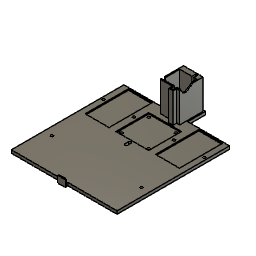
RobotBase (Autodesk Fusion 360 design; units mm, degrees)
Autodesk Fusion 360 part; units mm, degrees
sketch "Sketch2" plane through (0, 0, 0) normal (1, 0, 0) x (0, 0, -1)
  line L0 (0, 0) -> (0, 10)
  dimension "d53" = 10
  constraint coincident L0.start origin
  constraint vertical L0
  measures "d53" distance of L0.start L0.end
sketch "Sketch1" plane through (0, 0, 0) normal (0, 1, 0) x (1, 0, 0)
  line L0 (0, 0) -> (141.9, 0)
  line L1 (141.9, 0) -> (141.9, 151.05)
  line L2 (0, 151.05) -> (0, 0)
  line L3 (130.925, 43.6) -> (10.975, 43.6) construction
  circle A0 centre (10.975, 43.6) radius 1.75
  circle A1 centre (130.925, 43.6) radius 1.75
  line L4 (70.95, 0) -> (70.95, 43.6) construction
  line L5 (65.95, 0) -> (68.5, 0)
  line L6 (70.95, -2) -> (65.95, -2)
  line L7 (65.95, -2) -> (65.95, 0)
  line L8 (75.95, -2) -> (75.95, 0)
  line L9 (70.95, -2) -> (75.95, -2)
  line L10 (70.95, 43.6) -> (70.95, 85.6) construction
  line L11 (72.7, 88.1) -> (72.7, 83.1)
  line L12 (69.2, 83.1) -> (69.2, 88.1)
  arc A2 (72.7, 88.1) -> (69.2, 88.1) centre (70.95, 88.1) ccw
  arc A3 (69.2, 83.1) -> (72.7, 83.1) centre (70.95, 83.1) ccw
  line L13 (69.2, 85.6) -> (72.7, 85.6) construction
  line L14 (3.35, 120.45) -> (44.05, 120.45) construction
  circle A4 centre (3.35, 120.45) radius 1.75
  circle A5 centre (44.05, 120.45) radius 1.75
  line L15 (23.7, 151.05) -> (23.7, 120.45) construction
  line L16 (7.7, 149.45) -> (39.7, 149.45)
  line L17 (39.7, 149.45) -> (39.7, 91.45)
  line L18 (39.7, 91.45) -> (7.7, 91.45)
  line L19 (7.7, 91.45) -> (7.7, 149.45)
  line L20 (134.2, 91.45) -> (134.2, 149.45)
  line L21 (134.2, 149.45) -> (102.2, 149.45)
  line L22 (102.2, 149.45) -> (102.2, 91.45)
  circle A6 centre (138.55, 120.45) radius 1.75
  line L23 (102.2, 91.45) -> (134.2, 91.45)
  circle A7 centre (97.85, 120.45) radius 1.75
  line L24 (48.95, 135.45) -> (92.95, 135.45)
  line L25 (92.95, 135.45) -> (92.95, 91.45)
  line L26 (92.95, 91.45) -> (48.95, 91.45)
  line L27 (48.95, 91.45) -> (48.95, 135.45)
  line L28 (48.95, 113.45) -> (39.7, 113.45) construction
  line L29 (92.95, 113.45) -> (102.2, 113.45) construction
  circle A8 centre (52.7, 131.7) radius 1.75
  circle A9 centre (52.7, 95.2) radius 1.75
  circle A10 centre (89.2, 95.2) radius 1.75
  circle A11 centre (89.2, 131.7) radius 1.75
  line L30 (74.1, 142.05) -> (74.1, 137.05)
  line L31 (74.1, 173.25) -> (74.1, 168.25)
  line L32 (82.45, 143.65) -> (82.45, 166.65)
  line L33 (74.1, 173.25) -> (79.95, 173.25)
  line L34 (57.85, 142.05) -> (74.1, 142.05)
  line L35 (74.1, 168.25) -> (57.85, 168.25)
  line L36 (57.85, 142.05) -> (57.85, 168.25)
  line L37 (78.35, 138.65) -> (78.35, 143.65)
  line L38 (78.35, 166.65) -> (78.35, 171.65)
  line L39 (82.45, 166.65) -> (78.35, 166.65)
  line L40 (78.35, 143.65) -> (82.45, 143.65)
  line L41 (75.7, 166.65) -> (59.45, 166.65)
  line L42 (59.45, 166.65) -> (59.45, 143.65)
  line L43 (75.7, 171.65) -> (75.7, 166.65)
  line L44 (59.45, 143.65) -> (75.7, 143.65)
  line L45 (78.35, 171.65) -> (75.7, 171.65)
  line L46 (75.7, 138.65) -> (78.35, 138.65)
  line L47 (75.7, 143.65) -> (75.7, 138.65)
  line L48 (84.05, 142.05) -> (79.95, 142.05)
  line L49 (79.95, 137.05) -> (74.1, 137.05)
  line L50 (84.05, 168.25) -> (84.05, 142.05)
  line L51 (79.95, 142.05) -> (79.95, 137.05)
  line L52 (79.95, 168.25) -> (79.95, 173.25)
  line L53 (84.05, 168.25) -> (79.95, 168.25)
  line L54 (82.45, 155.15) -> (59.45, 155.15) construction
  line L55 (70.95, 155.15) -> (70.95, 135.45) construction
  line L56 (56.25, 151.05) -> (56.25, 174.85)
  line L57 (56.25, 174.85) -> (85.65, 174.85)
  line L58 (85.65, 174.85) -> (85.65, 151.05)
  line L59 (141.9, 151.05) -> (85.65, 151.05)
  line L60 (56.25, 151.05) -> (0, 151.05)
  line L61 (59.45, 143.65) -> (57.85, 143.65)
  line L62 (59.45, 147.65) -> (57.85, 147.65)
  line L63 (74.1, 173.25) -> (57.85, 173.25)
  line L64 (57.85, 173.25) -> (57.85, 168.25)
  line L65 (79.95, 173.25) -> (84.05, 173.25)
  line L66 (84.05, 173.25) -> (84.05, 168.25)
  line L67 (75.95, -2) -> (75.95, -3.6)
  line L68 (75.95, -3.6) -> (65.95, -3.6)
  line L69 (65.95, -3.6) -> (65.95, -2)
  point P0 (70.95, 113.45)
  point P1 (-289, 70)
  dimension "d1" = 141.9
  dimension "d2" = 151.05
  dimension "d3" = 119.95
  dimension "d4" = 3.5
  dimension "d6" = 5
  dimension "d8" = 43.6
  dimension "d9" = 42
  dimension "d10" = 3.5
  dimension "d11" = 5
  dimension "d12" = 40.7
  dimension "d13" = 3.5
  dimension "d14" = 3.35
  dimension "d15" = 30.6
  dimension "d16" = 58
  dimension "d17" = 1.6
  dimension "d18" = 32
  dimension "d19" = 16
  dimension "d20" = 44
  dimension "d23" = 44
  dimension "d24" = 3.35
  dimension "d25" = 3.5
  dimension "d26" = 3.75
  dimension "d27" = 3.75
  dimension "d28" = 22
  dimension "d29" = 22
  dimension "d31" = 360
  dimension "d32" = 4.9
  dimension "d33" = 4.9
  dimension "d34" = 1.6
  dimension "d35" = 1.6
  dimension "d36" = 1.6
  dimension "d37" = 1.6
  dimension "d38" = 1.6
  dimension "d39" = 1.6
  dimension "d40" = 1.6
  dimension "d41" = 1.6
  dimension "d42" = 1.6
  dimension "d43" = 1.6
  dimension "d44" = 1.6
  dimension "d45" = 1.6
  dimension "d47" = 5
  dimension "d48" = 23
  dimension "d49" = 23
  dimension "d50" = 4.1
  dimension "d51" = 6.75
  dimension "d54" = 1.6
  dimension "d55" = 1.6
  dimension "d56" = 1.6
  dimension "d57" = 1.6
  dimension "d58" = 4
  dimension "d80" = 2
  dimension "d81" = 1.6
  constraint horizontal L0
  constraint vertical L1
  constraint horizontal L59
  constraint vertical L2
  constraint coincident L0.start L2.end
  constraint perpendicular L2 L3
  constraint coincident L3.end A0.centre
  constraint coincident L3.start A1.centre
  constraint equal A0 A1
  constraint midpoint L0 L4.start
  constraint midpoint L3 L4.end
  constraint vertical L4
  constraint horizontal L5
  constraint horizontal L6
  constraint vertical L7
  constraint coincident L0 L5.start
  constraint coincident L4 L6.start
  constraint symmetric L4 L5.start L8.end
  constraint symmetric L4 L6.end L8.start
  constraint symmetric L4 L6.start L9.start
  constraint perpendicular L3 L10
  constraint vertical L11
  constraint vertical L12
  constraint tangent L12 A2
  constraint tangent L12 A3
  constraint tangent L11 A3
  constraint tangent L11 A2
  constraint coincident L10 A3.centre
  constraint midpoint L12 L13.start
  constraint midpoint L11 L13.end
  constraint coincident L10.end L13
  constraint horizontal L14
  constraint coincident L14.start A4.centre
  constraint coincident L14.end A5.centre
  constraint equal A4 A5
  constraint coincident L15.start L59
  constraint midpoint L14 L15.end
  constraint vertical L15
  constraint horizontal L16
  constraint vertical L17
  constraint horizontal L18
  constraint vertical L19
  constraint symmetric L10 A4 A6
  constraint symmetric L10 A5 A7
  constraint symmetric L10 L16.start L20.end
  constraint symmetric L10 L16.end L21.end
  constraint symmetric L10 L17.end L22.end
  constraint symmetric L10 L18.end L20.start
  constraint horizontal L24
  constraint vertical L25
  constraint horizontal L26
  constraint vertical L27
  constraint collinear L18 L26
  constraint midpoint L27 L28.start
  constraint coincident L17 L28.end
  constraint perpendicular L17 L28
  constraint midpoint L25 L29.start
  constraint coincident L22 L29.end
  constraint perpendicular L22 L29
  constraint equal L28 L29
  constraint perpendicular L31 L33
  constraint perpendicular L35 L36
  constraint perpendicular L50 L53
  constraint perpendicular L33 L52
  constraint perpendicular L48 L50
  constraint perpendicular L49 L51
  constraint perpendicular L34 L36
  constraint perpendicular L30 L49
  constraint coincident L32.start L40.end
  constraint collinear L37 L38
  constraint collinear L43 L47
  constraint collinear L40 L44
  constraint collinear L39 L41
  constraint equal L43 L47
  constraint midpoint L32 L54.start
  constraint midpoint L42 L54.end
  constraint midpoint L54 L55.start
  constraint midpoint L24 L55.end
  constraint perpendicular L54 L55
  constraint vertical L55
  constraint vertical L56
  constraint horizontal L57
  constraint vertical L58
  constraint collinear L59 L60
  constraint coincident L36 L61.end
  constraint perpendicular L36 L61
  constraint coincident L42 L62.start
  constraint coincident L36 L62.end
  constraint perpendicular L36 L62
  constraint perpendicular L36 L63
  constraint perpendicular L53 L64
  constraint perpendicular L50 L65
  constraint perpendicular L53 L66
  constraint vertical L67
  constraint horizontal L68
  constraint vertical L69
  constraint collinear L8 L67
  constraint coincident L8.start L9.end
  measures "d1" distance of L0.start L0.end
  measures "d2" distance of L0.start L2.start
  measures "d3" distance of L3.start L3.end
  measures "d4" diameter of A0
  measures "d6" distance of L6.end L6.start
  measures "d8" distance of L4.start L4.end
  measures "d9" distance of L4.end L10.end
  measures "d10" distance of L11 L12
  measures "d11" distance of L11.start L11.end
  measures "d12" distance of L14.start L14.end
  measures "d13" diameter of A4
  measures "d14" distance of L2 L14.start
  measures "d15" distance of L15.start L15.end
  measures "d16" distance of L16.start L18.end
  measures "d17" distance of L16 L59
  measures "d18" distance of L16.start L16.end
  measures "d19" distance of L15 L17
  measures "d20" distance of L24.start L24.end
  measures "d23" distance of L24.end L25.end
  measures "d24" distance of A2.centre L26
  measures "d25" diameter of A8
  measures "d26" distance of L27 A8.centre
  measures "d27" distance of L24 A8.centre
  measures "d28" distance of L29.start P0
  measures "d29" distance of L24 P0
  measures "d32" distance of A7.centre L25
  measures "d33" distance of L14.end L27
  measures "d34" distance of L33 L45
  measures "d35" distance of L36 L42
  measures "d36" distance of L46 L49
  measures "d37" distance of L37 L51
  measures "d38" distance of L40 L48
  measures "d39" distance of L39 L53
  measures "d40" distance of L38 L52
  measures "d41" distance of L31 L43
  measures "d42" distance of L35 L41
  measures "d43" distance of L30 L47
  measures "d44" distance of L34 L44
  measures "d45" distance of L32 L50
  measures "d47" distance of L44.end L46.start
  measures "d48" distance of L42.end L41.end
  measures "d49" distance of L32 L42
  measures "d50" distance of L32 L38
  measures "d51" distance of L32 L47
  measures "d54" distance of L24 L49
  measures "d55" distance of L50 L58
  measures "d56" distance of L36 L56
  measures "d57" distance of L33 L57
  measures "d58" distance of L61 L62
  measures "d80" distance of L0 L6
  measures "d81" distance of L6.end L68.end
extrude "Extrude1" add sketch "Sketch1" against normal blind 4 contours L0 L1 L2 L5 L56 L57 L58 L59 L60 | L0 L5 L6 L7 L8 L9 | L6 L9 L67 L68 L69 | L16 L17 L18 L19 | L20 L21 L22 L23 | L24 L25 L26 L27 | L30 L31 L32 L33 L34 L35 L36 L37 L38 L39 L40 L41 L42 L43 L44 L45 L46 L47 L48 L49 L50 L51 L52 L53 L61 L62 | L36 L42 L61 L62 | L32 L37 L38 L39 L40 L41 L42 L43 L44 L45 L46 L47 | L31 L35 L63 L64 | L52 L53 L65 L66
extrude "Extrude2" cut sketch "Sketch1" against normal blind 1.6 contours L16 L17 L18 L19 | L20 L21 L22 L23 | L24 L25 L26 L27
extrude "Extrude3" add sketch "Sketch1" along normal blind 5 contours L6 L9 L67 L68 L69
extrude "Extrude4" add sketch "Sketch1" along normal blind 40 contours L30 L31 L32 L33 L34 L35 L36 L37 L38 L39 L40 L41 L42 L43 L44 L45 L46 L47 L48 L49 L50 L51 L52 L53 L61 L62 | L31 L35 L63 L64 | L52 L53 L65 L66
sketch "Sketch3" plane through (84.05, 0, 0) normal (1, 0, 0) x (0, 0, -1)
  line L0 (142.05, 0) -> (173.25, 0)
  line L1 (173.25, 0) -> (173.25, 40)
  line L2 (173.25, 40) -> (142.05, 40)
  line L3 (142.05, 40) -> (142.05, 0)
  line L4 (143.65, 0) -> (143.65, 40)
  line L5 (155.65, 43) -> (154.8462, 43)
  line L6 (155.65, 37) -> (154.8462, 37)
  arc A0 (155.65, 37) -> (155.65, 43) centre (155.65, 40) ccw
  arc A1 (154.8462, 43) -> (154.8462, 37) centre (149.65, 40) ccw
  dimension "d69" = 6
  dimension "d70" = 12
  dimension "d71" = 6
  constraint tangent L4 A1
  constraint tangent L5 A0
  constraint horizontal L5
  constraint tangent L6 A0
  constraint parallel L5 L6
  constraint horizontal A1.centre A0.centre
  constraint coincident L2 A1.centre
  measures "d69" distance of A1.centre A0.centre
  measures "d70" diameter of A1
  measures "d71" diameter of A0
extrude "Extrude6" cut sketch "Sketch3" against normal blind 5 contours L2 L6 A0 A1
ref_plane "WorkPlane1" through (66.775, 20, -157.65) normal (0, 0, -1) x (-1, 0, 0)
sketch "Sketch4" plane through (66.775, 20, -157.65) normal (0, 0, -1) x (1, 0, 0)
  line L0 (-7.325, 20) -> (-7.325, -20)
  line L1 (-7.325, -20) -> (-7.325, 20)
  line L2 (-7.325, -5.5787) -> (-7.325, -0.4998)
  line L3 (8.925, 20) -> (-7.325, 20)
  line L4 (-7.325, -5.5787) -> (7.1393, 20)
  line L5 (-7.325, -0.4998) -> (4.2673, 20)
  line L6 (4.2673, 20) -> (7.1393, 20)
  dimension "d77" = 2.5
  constraint coincident L0 L2.start
  constraint coincident L0 L2.end
  constraint coincident L3 L5.end
  constraint parallel L4 L5
  constraint coincident L3 L4.end
  measures "d77" distance of L4 L5
extrude "Extrude7" add sketch "Sketch4" along normal mid plane 1.6 contours L0 L1 L2 L3 L4 L5 L6
equation "d15 = ( 58 / 2 ) * 1 mm + 1.6 mm"
equation "d34 = d44"
equation "d35 = d44"
equation "d36 = d44"
equation "d37 = d44"
equation "d38 = d44"
equation "d39 = d44"
equation "d40 = d44"
equation "d41 = d44"
equation "d42 = d44"
equation "d43 = d44"
equation "d45 = d44"
equation "d56 = d34"
equation "d57 = d55"
